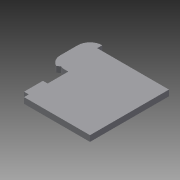
# Autodesk Inventor part: ExtruderSatoerMotorMount
Saved by Autodesk Inventor 2015 SP1 (Build 190203100, 203)
## iProperties
Created: 2015-05-03
Part Number: ExtruderSatoerMotorMount
Material: Generic
Document SubType Name: Modeling
Designer: Jack
Density: 1 g/cm^3
Appearance: Default
Author: Jack
Autodesk Inventor part; units mm, degrees
ref_plane "YZ Plane" through (0, 0, 0) normal (1, 0, 0) x (0, 1, 0)
ref_plane "XZ Plane" through (0, 0, 0) normal (0, 1, 0) x (-1, 0, 0)
ref_plane "XY Plane" through (0, 0, 0) normal (0, 0, 1) x (1, 0, 0)
sketch "Sketch1" plane through (0, 0, 0) normal (0, 0, 1) x (1, 0, 0)
  line L0 (0, 0) -> (45.5, 0)
  line L1 (45.5, 0) -> (45.5, 54.5)
  line L2 (0, 30.5) -> (-3, 30.5)
  line L3 (45.5, 54.5) -> (-4, 54.5)
  line L4 (-4, 54.5) -> (-4, 58)
  arc A0 (-5.6, 31.1534) -> (-3, 30.5) centre (-3, 36) ccw
  line L5 (-5.6, 31.1534) -> (-7.473, 29.7419)
  arc A1 (-12.5, 37.5) -> (-7.473, 29.7419) centre (-4, 37.5) ccw
  arc A2 (-4, 58) -> (-12.5, 49.5) centre (-4, 49.5) ccw
  line L6 (-12.5, 49.5) -> (-12.5, 37.5)
  line L7 (0, 0) -> (0, 3.25)
  line L8 (0, 3.25) -> (-3.25, 3.25)
  line L9 (-3.25, 3.25) -> (-3.25, 16.25)
  line L10 (-3.25, 16.25) -> (0, 16.25)
  line L11 (0, 16.25) -> (0, 30.5)
  dimension "d0" = 45.5
  dimension "d1" = 54.5
  dimension "d2" = 3.5
  dimension "d3" = 5.5
  dimension "d5" = 8.5
  dimension "d6" = 12
  dimension "d8" = 58
  dimension "d9" = 53
  dimension "d10" = 13
  dimension "d11" = 3.25
  dimension "d12" = 3.25
  dimension "d13" = 14.25
  dimension "d14" = 3
  dimension "d15" = 5.6
  constraints: 24 end point, 6 perpendicular, 6 point on circle, 3 centre point, 3 tangent, 2 horizontal, 2 vertical, 1 equal radius, 1 line through centre, 1 point on line, 1 vertical alignment
  measures "d0" distance of L0.start L0.end
  measures "d1" distance of L0.end L1.end
  measures "d2" distance of L3.end L4.end
  measures "d3" radius of A0
  measures "d5" radius of A2
  measures "d6" distance of A2.centre A1.centre
  measures "d8" distance between parallel lines of L1 L6
  measures "d9" angle of L6 L5
  measures "d10" distance of L8.end L9.end
  measures "d11" distance between parallel lines of L0 L8
  measures "d12" distance of L9.end L10.end
  measures "d13" distance of L10.end L2.start
  measures "d14" distance of L2.start L2.end
  measures "d15" horizontal distance of L2.start L5.start
extrude "Extrusion1" add sketch "Sketch1" along normal blind 4
body "Solid1"
